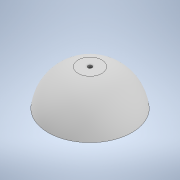
# Autodesk Inventor part: ball tops
Saved by Autodesk Inventor 2022 (Build 260153000, 153)
## iProperties
Created: 2022-03-14
Part Number: ball tops
Material: Generic
Document SubType Name: Modeling
Designer: mogje
Density: 1 g/cm^3
Appearance: Default
Author: mogje
Autodesk Inventor part; units mm, degrees
ref_plane "YZ Plane" through (0, 0, 0) normal (1, 0, 0) x (0, 1, 0)
ref_plane "XZ Plane" through (0, 0, 0) normal (0, 1, 0) x (-1, 0, 0)
ref_plane "XY Plane" through (0, 0, 0) normal (0, 0, 1) x (1, 0, 0)
sketch "Sketch1" plane through (0, 0, 0) normal (0, 1, 0) x (-1, 0, 0)
  arc A0 (-31.588, -3.2035) -> (31.588, 3.2035) centre (0, 0) ccw
  line L0 (0, 0) -> (-31.588, -3.2035) construction
  line L1 (0, 0) -> (31.588, 3.2035) construction
  line L2 (31.588, 3.2035) -> (-31.588, -3.2035)
  constraints: 6 end point, 3 point on circle, 1 centre point, 1 coincident
revolve "Revolution1" add sketch "Sketch1" angle 180 about axis through (0, 0, 0) along (0.9948968, 0, -0.1008975)
sketch "Sketch2" plane through (0, 0, 0) normal (0, -1, 0) x (1, 0, 0)
  circle A0 centre (0, 0) radius 31.75
  constraints: 1 centre point, 1 coincident
extrude "Extrusion1" cut sketch "Sketch2" against normal blind 30.48 keep common part
sketch "Sketch3" plane through (0, 0, 0) normal (0, -1, 0) x (1, 0, 0)
  line L0 (0, 0) -> (0, -27.94)
  circle A0 centre (0, 0) radius 8.89 projected
  line L1 (0, 0) -> (0, 25.4)
  circle A1 centre (0, 0) radius 27.94
  circle A2 centre (0, 0) radius 25.4
  dimension "d7" = 27.94
  dimension "d8" = 25.4
  constraints: 4 end point, 2 coincident, 2 vertical, 2 vertical alignment, 4 other
  measures "d7" distance of L0.start L0.end
  measures "d8" distance of L1.start L1.end
extrude "Extrusion2" cut sketch "Sketch3" against normal blind 3.175
sketch "Sketch4" plane through (0, 30.48, 0) normal (0, 1, 0) x (1, 0, 0)
  circle A0 centre (0, 0) radius 1.5875
  dimension "d11" = 3.175
  constraints: 1 centre point, 1 coincident
  measures "d11" diameter of A0
extrude "Extrusion3" cut sketch "Sketch4" against normal blind 6.35
sketch "Sketch5" plane through (0, 0, 0) normal (0, -1, 0) x (1, 0, 0)
  circle A0 centre (0, 0) radius 1.5875 projected
  circle A1 centre (0, 0) radius 31.75
  circle A2 centre (0, 0) radius 27.94
  constraints: 2 centre point, 2 coincident
extrude "Extrusion4" cut sketch "Sketch5" against normal blind 3.175 contours A1
body "Solid1"
